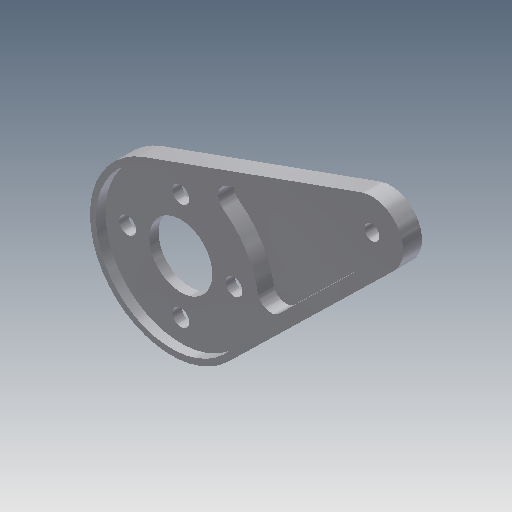
# Autodesk Inventor part: 足首_独立ピッチ_1_1
Saved by Autodesk Inventor 2017.3 (Build 213256000, 256)
## iProperties
Created: 2016-04-29
Part Number: 足首_独立ピッチ_1_1
Material: アルミニウム 2014-T4
Document SubType Name: Modeling
Designer: hiroaki
Density: 2.8 g/cm^3
Appearance: サテン
Mass: 4.32652 g
Surface Area: 25.7721 cm^2
Volume: 1.54518 cm^3
Author: hiroaki
Autodesk Inventor part; units mm, degrees
ref_plane "YZ Plane" through (0, 0, 0) normal (1, 0, 0) x (0, 1, 0)
ref_plane "XZ Plane" through (0, 0, 0) normal (0, 1, 0) x (-1, 0, 0)
ref_plane "XY Plane" through (0, 0, 0) normal (0, 0, 1) x (1, 0, 0)
derived "下半身全体像_1_1.ipt"
sketch "スケッチ1" plane through (0, 0, 0) normal (0, 0, 1) x (1, 0, 0)
  circle A0 centre (0, 0) radius 10.5 construction
  line L0 (0, 0) -> (-12, 0) construction
  arc A1 (0, 16) -> (-12, 10.583) centre (0, 0) ccw construction
  arc A2 (-12, -10.583) -> (0, -16) centre (0, 0) ccw construction
  line L1 (0, 16) -> (39.5, 16) construction
  line L2 (39.5, 16) -> (39.5, -16) construction
  line L3 (39.5, -16) -> (0, -16) construction
  circle A3 centre (1, 13.5) radius 1.35
  circle A4 centre (1, -13.5) radius 1.35
  circle A5 centre (28, 13.5) radius 1.35
  circle A6 centre (28, -13.5) radius 1.35
  line L4 (1, 13.5) -> (1, -13.5) construction
  line L5 (1, -13.5) -> (28, -13.5) construction
  line L6 (1, 13.5) -> (28, 13.5) construction
  line L7 (28, 13.5) -> (28, -13.5) construction
  line L8 (0, 0) -> (1, 0) construction
  line L9 (32, 120) -> (32, 20) construction
  line L10 (0, 0) -> (0, 0) construction
  circle A7 centre (32, 120) radius 4.05
  line L11 (0, 140) -> (0, 40) construction
  circle A8 centre (0, 40) radius 4.05
  line L12 (0, 0) -> (0, -100) construction
  line L13 (32, 20) -> (32, -80) construction
  line L14 (0, 0) -> (0, 40) construction
  circle A9 centre (32, 20) radius 6.5 construction
  line L15 (32, 23.5218) -> (35.05, 21.7609) construction
  line L16 (35.05, 21.7609) -> (35.05, 18.2391) construction
  line L17 (35.05, 18.2391) -> (32, 16.4782) construction
  line L18 (32, 16.4782) -> (28.95, 18.2391) construction
  line L19 (28.95, 18.2391) -> (28.95, 21.7609) construction
  line L20 (28.95, 21.7609) -> (32, 23.5218) construction
  line L21 (21.5, 152) -> (61, 152) construction
  line L22 (61, 152) -> (61, 100.5) construction
  line L23 (61, 100.5) -> (21.5, 100.5) construction
  line L24 (21.5, 100.5) -> (21.5, 152) construction
  line L25 (21.5, 140) -> (61, 140) construction
  line L26 (16, 150.5) -> (66.5, 150.5) construction
  line L27 (66.5, 150.5) -> (66.5, 129.5) construction
  line L28 (66.5, 129.5) -> (16, 129.5) construction
  line L29 (16, 129.5) -> (16, 150.5) construction
  circle A10 centre (0, 140) radius 10.5 construction
  line L30 (-13.5, 139) -> (13.5, 139) construction
  line L31 (13.5, 139) -> (13.5, 112) construction
  line L32 (13.5, 112) -> (-13.5, 112) construction
  line L33 (-13.5, 112) -> (-13.5, 139) construction
  circle A11 centre (-13.5, 139) radius 1.35
  circle A12 centre (13.5, 139) radius 1.35
  circle A13 centre (-13.5, 112) radius 1.35
  circle A14 centre (13.5, 112) radius 1.35
  line L34 (-12, 10.583) -> (-12, -10.583) construction
  circle A15 centre (0, -100) radius 4.05 construction
  circle A16 centre (32, -80) radius 4.05 construction
  circle A17 centre (0, -100) radius 10.5 construction
  line L35 (32, -80) -> (0, -100) construction
  line L36 (45, -60.5) -> (77.5, -60.5) construction
  line L37 (77.5, -60.5) -> (77.5, -112) construction
  line L38 (77.5, -112) -> (45, -112) construction
  line L39 (45, -112) -> (45, -60.5) construction
  line L40 (45, -100) -> (77.5, -100) construction
  line L41 (39.5, -89.5) -> (83, -89.5) construction
  line L42 (83, -89.5) -> (83, -110.5) construction
  line L43 (83, -110.5) -> (39.5, -110.5) construction
  line L44 (39.5, -110.5) -> (39.5, -89.5) construction
  line L45 (1, -86.5) -> (28, -86.5) construction
  line L46 (28, -86.5) -> (28, -113.5) construction
  line L47 (28, -113.5) -> (1, -113.5) construction
  line L48 (1, -113.5) -> (1, -86.5) construction
  circle A18 centre (1, -86.5) radius 1.35
  circle A19 centre (1, -113.5) radius 1.35
  circle A20 centre (28, -113.5) radius 1.35
  circle A21 centre (28, -86.5) radius 1.35
  circle A22 centre (32, 20) radius 4.05
  circle A23 centre (32, 20) radius 4.05
  line L49 (10.583, 152) -> (-10.583, 152) construction
  line L50 (16, 140) -> (16, 100.5) construction
  line L51 (16, 100.5) -> (-16, 100.5) construction
  line L52 (-16, 100.5) -> (-16, 140) construction
  arc A24 (16, 140) -> (10.583, 152) centre (0, 140) ccw construction
  arc A25 (-10.583, 152) -> (-16, 140) centre (0, 140) ccw construction
  line L53 (-12, -89.417) -> (-12, -110.583) construction
  line L54 (0, -84) -> (39.5, -84) construction
  line L55 (39.5, -84) -> (39.5, -116) construction
  line L56 (39.5, -116) -> (0, -116) construction
  arc A26 (0, -84) -> (-12, -89.417) centre (0, -100) ccw construction
  arc A27 (-12, -110.583) -> (0, -116) centre (0, -100) ccw construction
  circle A28 centre (-8.5, 0) radius 1.35
  circle A29 centre (0, 0) radius 8.5 construction
  line L57 (35.05, 121.7609) -> (35.05, 118.2391) construction
  line L58 (35.05, 118.2391) -> (32, 116.4782) construction
  line L59 (32, 116.4782) -> (28.95, 118.2391) construction
  line L60 (28.95, 118.2391) -> (28.95, 121.7609) construction
  line L61 (28.95, 121.7609) -> (32, 123.5218) construction
  line L62 (32, 123.5218) -> (35.05, 121.7609) construction
  circle A30 centre (32, -80) radius 1.2
  circle A31 centre (32, -80) radius 5 construction
  circle A32 centre (0, -100) radius 5.05
  circle A33 centre (-8.5, -100) radius 1.35
  circle A34 centre (0, -108.5) radius 1.35
  circle A35 centre (8.5, -100) radius 1.35
  circle A36 centre (0, -91.5) radius 1.35
  line L63 (9.0705, -109.3127) -> (35.4886, -83.5818)
  arc A37 (-4.3963, -87.7659) -> (9.0705, -109.3127) centre (0, -100) ccw
  line L64 (0, 152) -> (0, 140) construction
  line L65 (0, 140) -> (0, 139) construction
  line L66 (-4.3963, -87.7659) -> (30.3091, -75.2946)
  arc A38 (35.4886, -83.5818) -> (30.3091, -75.2946) centre (32, -80) ccw
  circle A39 centre (-8.5, -100) radius 2.5 construction
  circle A40 centre (0, -100) radius 11 construction
  circle A41 centre (0, -100) radius 12 construction
  point P0 (66.5, 140)
  point P1 (39.5, 0)
  point P2 (83, -100)
  point P3 (1, -100)
  point P4 (-12, -100)
  point P5 (39.5, -100)
  dimension "d5" = 17
  dimension "d3" = 10.1
  dimension "d4" = 2.7
  dimension "d6" = 8.5
  dimension "d9" = 360
  dimension "d13" = 10
  dimension "d14" = 2.4
  dimension "d21" = 5
  dimension "d22" = 1
  dimension "d23" = 1
  measures "d3" diameter of A32
  measures "d4" diameter of A33
  measures "d6" distance of A26.centre A33.centre
  measures "d13" diameter of A31
  measures "d14" diameter of A30
  measures "d21" diameter of A39
  measures "d22" radial gap between concentric circles of A41 A40
  measures "d23" radial gap between concentric circles of A37 A41
extrude "押し出し1" add sketch "スケッチ1" along normal blind 3 contours A18 L66 | A18 L66 A38 L63 A37 A19 | A19 A37 | A21 picked at (1.0956, -86.821) picked at (0.9957, -112.6894)
sketch "スケッチ3" plane through (9.0705, -109.3127, 3) normal (0, 0, 1) x (0.7163635, 0.6977272, 0)
  circle A0 centre (0, 13) radius 5.05 projected
  circle A1 centre (5.9307, 19.0891) radius 1.35 projected
  circle A2 centre (6.0891, 7.0693) radius 1.35 projected
  circle A3 centre (-5.9307, 6.9109) radius 1.35 projected
  circle A4 centre (-6.0891, 18.9307) radius 1.35 projected
  arc A5 (5.3867, 24.8315) -> (0, 0) centre (0, 13) ccw projected
  circle A6 centre (0, 13) radius 12 construction
  circle A7 centre (0, 13) radius 12.05
  point P0 (69.7727, 84.6364)
  dimension "d17" = 0.05
  dimension "d19" = 24
  constraints: 2 centre point, 1 coincident
  measures "d17" radial gap between concentric circles of A7 A6
  measures "d19" diameter of A6
extrude "押し出し2" cut sketch "スケッチ3" against normal blind 1.5
sketch "スケッチ4" plane through (0, -100, 3) normal (0, 0, 1) x (0.8479983, 0.5299989, 0)
  circle A0 centre (0, 0) radius 12.05 projected
  circle A1 centre (37.7359, 0) radius 1.2 projected
  line L0 (2.756, -12.7045) -> (38.7959, -4.8863) projected
  arc A2 (38.7959, -4.8863) -> (38.7959, 4.8863) centre (37.7359, 0) ccw projected
  line L1 (38.7959, 4.8863) -> (2.756, 12.7045) projected
  circle A3 centre (37.7359, 0) radius 5 construction
  arc A4 (34.4628, 3.7798) -> (34.4628, -3.7798) centre (37.7359, 0) ccw
  line L2 (34.4628, -3.7798) -> (10.8742, -8.8969)
  line L3 (34.4628, 3.7798) -> (10.8742, 8.8969)
  arc A5 (10.8742, -8.8969) -> (10.8742, 8.8969) centre (0, 0) ccw
  point P0 (52.9999, 84.7998)
  dimension "d24" = 2
  dimension "d25" = 2
  dimension "d26" = 2
  constraints: 4 end point, 4 point on circle, 3 centre point, 3 coincident, 2 concentric, 2 parallel
  measures "d24" radial gap between concentric circles of A0 A5
  measures "d25" distance between parallel lines of L0 L2
  measures "d26" distance between parallel lines of L1 L3
extrude "押し出し3" cut sketch "スケッチ4" against normal blind 2.5 contours A4 L2 A5 L3
fillet "フィレット2" radius 2 4 edges at (31.2277, -84.94, 1.75) (27.2211, -78.5295, 1.75) (13.9366, -101.7813, 1.75) (4.5059, -86.6921, 1.75)
equation "\"d6\" = 0.5 * d5"
equation "\"d26\" = d25"
